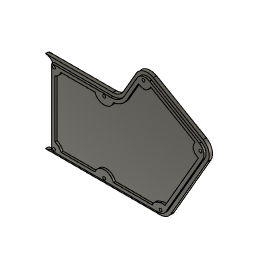
Barcode+scanner (Autodesk Fusion 360 design; units mm, degrees)
Autodesk Fusion 360 part; units mm, degrees
(part 1 of 5)
sketch "Sketch1" plane through (0, 0, 0) normal (0, 1, 0) x (1, 0, 0) in component "GM60 standalone"
  line L0 (0, 0) -> (165.7543, 0)
  line L1 (178.7446, -7.5) -> (207.1218, -56.6506)
  line L2 (201.6314, -77.141) -> (166.9904, -97.141)
  line L3 (146.5, -91.6506) -> (138.3301, -77.5)
  line L4 (125.3397, -70) -> (19, -70)
  line L5 (4, -85) -> (4, -112)
  line L6 (1, -115) -> (0, -115)
  line L7 (0, -115) -> (0, 0)
  arc A0 (178.7446, -7.5) -> (165.7543, 0) centre (165.7543, -15) ccw
  arc A1 (201.6314, -77.141) -> (207.1218, -56.6506) centre (194.1314, -64.1506) ccw
  arc A2 (146.5, -91.6506) -> (166.9904, -97.141) centre (159.4904, -84.1506) ccw
  arc A3 (138.3301, -77.5) -> (125.3397, -70) centre (125.3397, -85) ccw
  arc A4 (19, -70) -> (4, -85) centre (19, -85) ccw
  line L8 (4, -4) -> (165.7543, -4)
  arc A5 (175.2805, -9.5) -> (165.7543, -4) centre (165.7543, -15) ccw
  line L9 (175.2805, -9.5) -> (203.6577, -58.6506)
  arc A6 (199.6314, -73.6769) -> (203.6577, -58.6506) centre (194.1314, -64.1506) ccw
  line L10 (199.6314, -73.6769) -> (164.9904, -93.6769)
  arc A7 (149.9641, -89.6506) -> (164.9904, -93.6769) centre (159.4904, -84.1506) ccw
  line L11 (149.9641, -89.6506) -> (141.7942, -75.5)
  arc A8 (141.7942, -75.5) -> (125.3397, -66) centre (125.3397, -85) ccw
  line L12 (125.3397, -66) -> (19, -66)
  arc A9 (19, -66) -> (4, -73.3381) centre (19, -85) ccw
  line L13 (4, -73.3381) -> (4, -4)
  arc A10 (1, -115) -> (4, -112) centre (1, -112) ccw
  arc A11 (4, -14) -> (14, -4) centre (4, -4) ccw
  line L14 (4, -4) -> (11.0711, -11.0711) construction
  circle A12 centre (7.5355, -7.5355) radius 2
  line L15 (19, -85) -> (19, -51) construction
  arc A13 (4, -51) -> (19, -66) centre (19, -51) ccw
  line L16 (19, -66) -> (4, -66) construction
  circle A14 centre (7, -66) radius 2
  line L17 (159.4904, -84.1506) -> (154, -104.641) construction
  spline S0 degree 2 poles (149.9641, -89.6506) (159.4904, -84.1506) (164.9904, -93.6769) knots 0 0 0 1.944544 1.944544 1.944544 weights 1 3 1
  circle A15 centre (157.6786, -90.9121) radius 2
  line L18 (175.2805, -9.5) -> (172.1601, -11.3016)
  line L19 (162.6789, -4) -> (162.6789, -6.8969)
  line L20 (164.656, -9.7171) -> (169.6373, -11.5237)
  arc A16 (162.6789, -6.8969) -> (164.656, -9.7171) centre (165.6789, -6.8969) ccw
  arc A17 (169.6373, -11.5237) -> (172.1601, -11.3016) centre (170.6601, -8.7035) ccw
  spline S1 degree 2 poles (199.6314, -73.6769) (194.1314, -64.1506) (203.6577, -58.6506) knots 0 0 0 1.944543 1.944543 1.944543 weights 1 3 1
  line L21 (194.1314, -64.1506) -> (214.6218, -69.641) construction
  circle A18 centre (200.8929, -65.9624) radius 2
  line L22 (162.6789, -4) -> (175.2805, -9.5) construction
  arc A19 (125.3397, -66) -> (109.3397, -66) centre (117.3397, -66) ccw
  line L23 (117.3397, -66) -> (117.3397, -58) construction
  circle A20 centre (117.3397, -62) radius 2
  line L24 (4, -85) -> (0, -85)
  line L25 (168.9797, -6.75) -> (167.1467, -10.6204) construction
  circle A21 centre (168.5515, -7.6542) radius 2
  circle A22 centre (7.5355, -7.5355) radius 2.25
  circle A23 centre (168.5515, -7.6542) radius 2.25
  circle A24 centre (200.8929, -65.9624) radius 2.25
  circle A25 centre (117.3397, -62) radius 2.25
  circle A26 centre (7, -66) radius 2.25
  circle A27 centre (157.6786, -90.9121) radius 2.25
  line L26 (4, -38.669) -> (192.1213, -38.669) construction
  line L27 (157, -6.669) -> (87, -6.669)
  line L28 (87, -6.669) -> (87, -56.669)
  line L29 (87, -56.669) -> (157, -56.669)
  line L30 (157, -56.669) -> (157, -6.669)
  line L31 (157, -6.669) -> (87, -56.669) construction
  line L32 (87, -6.669) -> (157, -56.669) construction
  line L33 (155.04, -8.604) -> (88.96, -8.604)
  line L34 (88.96, -8.604) -> (88.96, -54.734) construction
  line L35 (88.96, -54.734) -> (155.04, -54.734) construction
  line L36 (155.04, -54.734) -> (155.04, -8.604) construction
  line L37 (155.04, -8.604) -> (88.96, -54.734) construction
  line L38 (88.96, -8.604) -> (155.04, -54.734) construction
  circle A28 centre (88.96, -54.734) radius 0.95
  circle A29 centre (88.96, -54.734) radius 3.45
  circle A30 centre (155.04, -54.734) radius 0.95
  circle A31 centre (155.04, -54.734) radius 3.45
  circle A32 centre (155.04, -8.604) radius 0.95
  circle A33 centre (155.04, -8.604) radius 3.45
  circle A34 centre (88.96, -8.604) radius 3.45
  circle A35 centre (88.96, -8.604) radius 0.95
  point P0 (214.6218, -69.641)
  point P1 (154, -104.641)
  point P2 (134, -70)
  point P3 (4, -70)
  point P4 (4, -115)
  point P5 (170.9504, -12)
  point P6 (162.6789, -9)
  point P7 (122, -31.669)
  point P8 (122, -31.669)
  point P9 (122, -31.669)
  dimension "d1" = 130
  dimension "d2" = 70
  dimension "d3" = 70
  dimension "d4" = 40
  dimension "d5" = 4
  dimension "d7" = 45
  dimension "d8" = 120
  dimension "d9" = 4
  dimension "d40" = 15
  dimension "d47" = 3
  dimension "d84" = 10
  dimension "d85" = 4
  dimension "d88" = 19
  dimension "d94" = 15
  dimension "d95" = 19
  dimension "d96" = 15
  dimension "d97" = 15
  dimension "d98" = 3
  dimension "d101" = 11
  dimension "d102" = 15
  dimension "d105" = 7
  dimension "d111" = 5
  dimension "d112" = 5
  dimension "d113" = 3
  dimension "d115" = 7
  dimension "d120" = 8
  dimension "d121" = 8
  dimension "d139" = 1
  dimension "d147" = 0.25
  dimension "d148" = 0.25
  dimension "d149" = 0.25
  dimension "d150" = 0.25
  dimension "d151" = 0.25
  dimension "d153" = 3.2821
  dimension "d157" = 0.25
  dimension "d234" = 70
  dimension "d235" = 50
  dimension "d236" = 66.08
  dimension "d237" = 46.13
  dimension "d238" = 1.9
  dimension "d239" = 2.5
  dimension "d240" = 7
  dimension "d241" = 118
  constraint coincident L0.start L7.end
  constraint horizontal L0
  constraint perpendicular L1 L2
  constraint parallel L0 L4
  constraint perpendicular L4 L5
  constraint parallel L1 L3
  constraint perpendicular L5 L6
  constraint perpendicular L0 L7
  constraint tangent L0 A0
  constraint tangent L1 A0
  constraint coincident P0 L1
  constraint coincident P0 L2
  constraint tangent L1 A1
  constraint tangent L2 A1
  constraint equal A0 A1
  constraint coincident P1 L2
  constraint coincident P1 L3
  constraint tangent L2 A2
  constraint tangent L3 A2
  constraint equal A0 A2
  constraint coincident P2 L3
  constraint coincident P2 L4
  constraint tangent L3 A3
  constraint tangent L4 A3
  constraint equal A0 A3
  constraint coincident P3 L4
  constraint coincident P3 L5
  constraint tangent L4 A4
  constraint tangent L5 A4
  constraint equal A0 A4
  constraint coincident P4 L5
  constraint coincident P4 L6
  constraint tangent L5 A10
  constraint tangent L6 A10
  constraint coincident L13 A11.start
  constraint coincident L8 A11.end
  constraint coincident L8.start L13.end
  constraint midpoint A11 L14.end
  constraint midpoint L14 A12.centre
  constraint coincident A4.centre A9.centre
  constraint perpendicular L12 L15
  constraint coincident L13 A13.start
  constraint coincident L15.end A13.centre
  constraint coincident L13 L16.end
  constraint tangent A9 L16
  constraint perpendicular L13 L16
  constraint coincident L16 A14.centre
  constraint equal A12 A14
  constraint coincident A2.centre A7.centre
  constraint coincident P1 L17.end
  constraint coincident L17 A15.centre
  constraint equal A12 A15
  constraint perpendicular L9 L18
  constraint coincident L8 L19.start
  constraint perpendicular L8 L19
  constraint coincident P6 L19
  constraint coincident P6 L20
  constraint tangent L19 A16
  constraint tangent L20 A16
  constraint coincident P5 L20
  constraint coincident P5 L18
  constraint tangent L20 A17
  constraint tangent L18 A17
  constraint equal A16 A17
  constraint coincident A1.centre A6.centre
  constraint coincident P0 L21.end
  constraint coincident L21 A18.centre
  constraint equal A12 A18
  constraint coincident L12 A8.end
  constraint coincident L12 A19.centre
  constraint coincident A19.centre L23.start
  constraint perpendicular L12 L23
  constraint midpoint L23 A20.centre
  constraint equal A12 A20
  constraint coincident L7 L24.end
  constraint perpendicular L7 L24
  constraint midpoint L22 L25.start
  constraint midpoint L20 L25.end
  constraint coincident L25 A21.centre
  constraint equal A12 A21
  constraint midpoint L13 L26.start
  constraint coincident L9 L26.end
  constraint perpendicular L13 L26
  constraint horizontal L27
  constraint perpendicular L27 L28
  constraint parallel L27 L29
  constraint parallel L28 L30
  constraint coincident L31 P9
  constraint coincident L32 P9
  constraint coincident P9 P8
  constraint horizontal L33
  constraint perpendicular L33 L34
  constraint parallel L33 L35
  constraint parallel L34 L36
  constraint coincident L37 P9
  constraint coincident L38 P9
  constraint coincident L34.end L35.start
  constraint coincident L35.end L36.start
  constraint coincident L33.start L36.end
  constraint concentric A32 A33
  constraint coincident L33.end L34.start
  constraint concentric A34 A35
  constraint equal A29 A31
  constraint equal A31 A33
  constraint equal A33 A34
  constraint equal A28 A32
  constraint equal A30 A32
  constraint equal A30 A35
  measures "d1" distance of P2 P3
  measures "d2" distance of L0 L4
  measures "d3" distance of P0 P1
  measures "d4" distance of P1 P2
  measures "d5" distance of P4 L6.end
  measures "d7" distance of P3 P4
  measures "d8" angle of L3 L4
  measures "d40" radius of A0
  measures "d47" radius of A10
  measures "d84" radius of A11
  measures "d85" diameter of A12
  measures "d88" radius of A9
  measures "d94" distance of L4.end A4.centre
  measures "d95" distance of A4.centre L12
  measures "d96" distance of L5.start A4.centre
  measures "d97" distance of L12.end L15.end
  measures "d98" distance of L13 A14.centre
  measures "d101" radius of A7
  measures "d102" radius of A2
  measures "d105" distance of A2.centre A15.centre
  measures "d111" distance of L19.start P6
  measures "d112" distance of A5.start P5
  measures "d113" radius of A16
  measures "d115" distance of A1.centre A18.centre
  measures "d120" radius of A19
  measures "d121" distance of A8.end A19.centre
  measures "d139" distance of L22 A21.centre
  measures "d153" distance of L25.end A21.centre
  measures "d234" distance of L28.end L29.end
  measures "d235" distance of L27.end L28.end
  measures "d236" distance of L34.end L35.end
  measures "d237" distance of L33.end L34.end
  measures "d238" diameter of A28
  measures "d240" distance of L26 P9
  measures "d241" distance of L13 P9
extrude "Extrude1" add sketch "Sketch1" along normal blind 60 contours L0 L1 L2 L3 L4 L7 A0 A1 A2 A3 A4 L24 | L5 L6 L7 A10 L24 picked at (59.9181, -1.3333) picked at (1.3333, -104) makes body 1 in component "GM60 standalone"
sketch "Display cutout" plane through (81.8109, 0, 141.7006) normal (-0.5, 0, -0.866025) x (0, -1, 0) in component "GM60 standalone"
  line L0 (0, -136.0474) -> (0, -96.0474)
  line L1 (-60, -96.0474) -> (-60, -136.0474)
  line L2 (0, -116.0474) -> (-60, -116.0474) construction
  line L3 (0, -96.0474) -> (-60, -96.0474)
  line L4 (-60, -136.0474) -> (0, -136.0474)
  line L5 (-38.325, -103.0474) -> (-38.325, -108.5474)
  line L6 (-43.825, -123.5474) -> (-43.825, -132.5474)
  line L7 (-43.825, -103.0474) -> (-16.175, -103.0474)
  line L8 (-43.825, -132.5474) -> (-43.825, -127.8474)
  line L9 (-43.825, -132.5474) -> (-16.175, -132.5474)
  line L10 (-38.325, -132.5474) -> (-43.825, -132.5474)
  line L11 (-43.825, -127.8474) -> (-38.325, -127.8474)
  line L12 (-38.325, -127.8474) -> (-38.325, -132.5474)
  line L13 (-43.825, -108.5474) -> (-43.825, -103.0474)
  line L14 (-43.825, -108.5474) -> (-43.825, -123.5474)
  line L15 (-16.175, -123.5474) -> (-16.175, -108.5474)
  line L16 (-21.675, -132.5474) -> (-21.675, -127.8474)
  line L17 (-43.825, -123.5474) -> (-16.175, -108.5474) construction
  line L18 (-16.175, -103.0474) -> (-16.175, -108.5474)
  line L19 (-16.175, -132.5474) -> (-16.175, -123.5474)
  line L20 (-21.675, -127.8474) -> (-16.175, -127.8474)
  line L21 (-16.175, -127.8474) -> (-16.175, -132.5474)
  line L22 (-16.175, -108.5474) -> (-43.825, -108.5474)
  line L23 (-16.175, -123.5474) -> (-43.825, -123.5474)
  line L24 (-43.825, -123.5474) -> (-16.175, -123.5474)
  line L25 (-16.175, -108.5474) -> (-43.825, -108.5474)
  line L26 (-21.675, -103.0474) -> (-21.675, -108.5474)
  line L27 (-16.175, -123.5474) -> (-43.825, -108.5474) construction
  line L28 (-16.175, -132.5474) -> (-21.675, -132.5474)
  point P0 (-30, -116.0474)
  point P1 (-30, -116.0474)
  point P2 (-30, -116.0474)
  dimension "d64" = 27.65
  dimension "d65" = 15
  dimension "d66" = 5.5
  dimension "d67" = 9
  dimension "d68" = 5.5
  dimension "d69" = 5.5
  dimension "d70" = 4.7
  dimension "d225" = 29.5
  dimension "d226" = 24.8
  constraint midpoint L0 L2.start
  constraint midpoint L1 L2.end
  constraint horizontal L24
  constraint perpendicular L15 L24
  constraint parallel L24 L25
  constraint parallel L14 L15
  constraint coincident P2 L17
  constraint coincident P2 L27
  constraint perpendicular L13 L22
  constraint parallel L7 L22
  constraint parallel L13 L18
  constraint perpendicular L6 L23
  constraint parallel L9 L23
  constraint parallel L6 L19
  constraint coincident L26.start L7
  constraint coincident L26.end L25
  constraint perpendicular L25 L26
  constraint coincident L5.start L7
  constraint coincident L5.end L22
  constraint perpendicular L5 L22
  constraint horizontal L28
  constraint vertical L16
  constraint horizontal L20
  constraint vertical L21
  constraint collinear L16 L26
  constraint horizontal L10
  constraint vertical L8
  constraint horizontal L11
  constraint vertical L12
  constraint coincident L8.end L6
  constraint coincident L10.start L9
  constraint collinear L5 L12
  constraint collinear L11 L20
  constraint coincident P2 P1
  constraint midpoint L2 P2
  measures "d64" distance of L15.end L13.start
  measures "d65" distance of L15.end L15.start
  measures "d66" distance of L15.end L7.end
  measures "d67" distance of L15.start L9.end
  measures "d68" distance of L18 L26
  measures "d69" distance of L5 L13
  measures "d70" distance of L20 L28
  measures "d225" distance of L7 L9
  measures "d226" distance of L7 L20
sketch "Sketch1 (2)" plane through (0, 0, 0) normal (0, 0, 1) x (1, 0, 0) in component "Sample display"
  line L0 (9.6502, -9.1979) -> (15.1502, -9.1979)
  line L1 (-12.4998, -13.8979) -> (-12.4998, -9.1979)
  line L2 (-12.4998, 10.1021) -> (-12.4998, 15.6021)
  line L3 (-6.9998, -9.1979) -> (-6.9998, -13.8979)
  line L4 (15.1502, -4.8979) -> (-12.4998, -4.8979)
  line L5 (-12.4998, -4.8979) -> (15.1502, 10.1021) construction
  line L6 (9.6502, -13.8979) -> (9.6502, -9.1979)
  line L7 (-6.9998, 15.6021) -> (-6.9998, 10.1021)
  line L8 (-6.9998, -13.8979) -> (-12.4998, -13.8979)
  line L9 (-12.4998, -4.8979) -> (-12.4998, -13.8979)
  line L10 (9.6502, 15.6021) -> (9.6502, 10.1021)
  line L11 (15.1502, -4.8979) -> (15.1502, 10.1021)
  line L12 (15.1502, 10.1021) -> (-12.4998, 10.1021)
  line L13 (15.1502, -13.8979) -> (15.1502, -4.8979)
  line L14 (-12.4998, -9.1979) -> (-6.9998, -9.1979)
  line L15 (15.1502, -13.8979) -> (9.6502, -13.8979)
  line L16 (15.1502, 10.1021) -> (-12.4998, 10.1021)
  line L17 (-12.4998, -13.8979) -> (15.1502, -13.8979)
  line L18 (-12.4998, -4.8979) -> (15.1502, -4.8979)
  line L19 (15.1502, -9.1979) -> (15.1502, -13.8979)
  line L20 (15.1502, 15.6021) -> (15.1502, 10.1021)
  line L21 (15.1502, -4.8979) -> (-12.4998, 10.1021) construction
  line L22 (-12.4998, 10.1021) -> (-12.4998, -4.8979)
  line L23 (30, 0.866) -> (-30, 0.866) construction
  line L24 (-12.4998, 15.6021) -> (15.1502, 15.6021)
  line L25 (21.1502, -19.8979) -> (-18.4998, -19.8979)
  line L26 (-18.4998, -19.8979) -> (-18.4998, 21.6021)
  line L27 (-18.4998, 21.6021) -> (21.1502, 21.6021)
  line L28 (21.1502, 21.6021) -> (21.1502, -19.8979)
  line L29 (21.1502, -19.8979) -> (-18.4998, 21.6021) construction
  line L30 (-18.4998, -19.8979) -> (21.1502, 21.6021) construction
  point P0 (1.3252, 2.6021)
  point P1 (1.3252, 0.8521)
  point P2 (1.3252, 2.6021)
  point P3 (0, 0.866)
  point P4 (1.3252, 0.8521)
  dimension "d202" = 27.65
  dimension "d203" = 15
  dimension "d204" = 5.5
  dimension "d205" = 9
  dimension "d206" = 5.5
  dimension "d207" = 5.5
  dimension "d208" = 4.7
  dimension "d211" = 6
  dimension "d212" = 6
  dimension "d213" = 6
  dimension "d214" = 6
  dimension "d221" = 29.5
  dimension "d224" = 24.8
  constraint coincident P3 L23
  constraint midpoint P3 L23
  constraint horizontal L18
  constraint perpendicular L11 L18
  constraint parallel L12 L18
  constraint parallel L11 L22
  constraint coincident P2 L5
  constraint coincident P2 L21
  constraint perpendicular L2 L16
  constraint parallel L16 L24
  constraint parallel L2 L20
  constraint perpendicular L4 L9
  constraint parallel L4 L17
  constraint parallel L9 L13
  constraint coincident L10.start L24
  constraint coincident L10.end L12
  constraint perpendicular L10 L12
  constraint coincident L7.start L24
  constraint coincident L7.end L16
  constraint perpendicular L7 L16
  constraint horizontal L15
  constraint vertical L6
  constraint horizontal L0
  constraint vertical L19
  constraint collinear L6 L10
  constraint horizontal L8
  constraint vertical L1
  constraint horizontal L14
  constraint vertical L3
  constraint coincident L1.end L9
  constraint coincident L3.end L17
  constraint collinear L3 L7
  constraint collinear L0 L14
  constraint coincident P2 P0
  constraint horizontal L25
  constraint perpendicular L25 L26
  constraint parallel L25 L27
  constraint parallel L26 L28
  constraint coincident L29 P4
  constraint coincident L30 P4
  constraint coincident P4 P1
  measures "d202" distance of L5.end L2.start
  measures "d203" distance of L5.end L4.start
  measures "d204" distance of L5.end L20.start
  measures "d205" distance of L13.start L4.start
  measures "d206" distance of L10 L20
  measures "d207" distance of L2 L7
  measures "d208" distance of L0 L15
  measures "d211" distance of L24 L27
  measures "d212" distance of L22 L26
  measures "d213" distance of L11 L28
  measures "d214" distance of L17 L25
  measures "d221" distance of L17 L24
  measures "d224" distance of L14 L24
extrude "Extrude1'" add sketch "Sketch1 (2)" along normal blind 4 separate body contours L25 L26 L27 L28 picked at (19.1502, -1.0645) makes body 2 in component "Sample display"
extrude "Extrude2" add sketch "Sketch1 (2)" along normal blind 0.6 contours L0 L3 L4 L6 L9 L13 L14 L17 L18 | L7 L10 L12 L16 L24 picked at (-1.4498, -6.3312) picked at (-1.4498, 13.7688) bodies 2 in component "Sample display"
extrude "Extrude3" add sketch "Sketch1 (2)" along normal blind 2 contours L0 L6 L13 L15 L17 L19 | L1 L3 L8 L9 L14 L17 | L10 L12 L16 L20 L24 | L2 L7 L12 L16 L24 picked at (13.3168, -10.7645) picked at (-8.8332, -10.7645) picked at (13.3168, 11.9355) picked at (-10.6665, 13.7688) bodies 2 in component "Sample display"
fillet "Fillet1" radius 15 4 edges at (-18.4998, 21.6021, 2) (21.1502, 21.6021, 2) (-18.4998, -19.8979, 2) (21.1502, -19.8979, 2) on bodies 2 in component "Sample display"
extrude "Extrude8" add sketch "Sketch1" against normal blind 4 contours L0 L1 L2 L3 L4 L7 A0 A1 A2 A3 A4 L24 | L5 L6 L7 A10 L24 | L8 L13 A11 | L8 L9 L10 L11 A8 L12 L13 A11 A13 S0 L18 L19 L20 A16 A17 S1 A19 | L8 A5 L18 L19 L20 A16 A17 | A9 L13 A13 | L12 A19 | A6 S1 | A7 S0 | A12 | A14 | A15 | A18 | A20 | A21 | A22 | A23 | A24 | A25 | A26 | A27 | L27 L30 A33 | L27 L30 A33 | L27 L33 A33 A34 | L28 L29 L30 L33 A29 A31 A33 A34 | L27 L28 A34 | L27 L28 A34 | L29 L30 A31 | L29 L30 A31 | L28 L29 A29 | L28 L29 A29 | A28 | A30 | A32 | A35 picked at (59.9181, -1.3333) picked at (1.3333, -104) picked at (4.4369, -8.6236) picked at (39.1305, -42.8013) picked at (172.3644, -9.3579) picked at (11.2568, -65.9119) picked at (117.2837, -65.4146) picked at (198.6139, -69.7182) picked at (153.9527, -88.5857) picked at (6.8451, -7.203) picked at (6.363, -67.1034) picked at (158.3157, -92.0155) picked at (201.5299, -67.0658) picked at (116.4591, -62.4828) picked at (168.3942, -8.8468) picked at (9.6938, -7.6473) picked at (170.7098, -7.766) picked at (198.7346, -66.0742) picked at (118.0242, -64.0499) picked at (7.0498, -68.1606) picked at (155.7826, -89.875) picked at (156.6598, -8.9526) picked at (153.8961, -6.5342) picked at (131.8633, -8.2629) picked at (132.0458, -38.7358) picked at (87.3402, -8.9526) picked at (90.1066, -6.5371) picked at (153.8961, -56.8039) picked at (156.6598, -54.3855) picked at (87.3402, -54.3855) picked at (90.1066, -56.801) picked at (89.1921, -54.9494) picked at (155.3016, -54.8305) picked at (155.3253, -8.7414) picked at (88.7279, -8.9138) bodies 1 in component "GM60 standalone"
sketch "Sensor cutout" plane through (0, 0, 66) normal (0, 0, -1) x (1, 0, 0) in component "GM60 standalone"
  line L0 (125.3397, 0) -> (19, 0)
  line L1 (19, 0) -> (19, -60)
  line L2 (19, -60) -> (125.3397, -60)
  line L3 (125.3397, -60) -> (125.3397, 0)
  line L4 (19, -30) -> (125.3397, -30) construction
  circle A0 centre (69, -30) radius 13
  dimension "d48" = 26
  dimension "d49" = 50
  constraint midpoint L1 L4.start
  constraint coincident L4 A0.centre
  measures "d48" diameter of A0
  measures "d49" distance of L4.start A0.centre
extrude "Extrude1''" cut sketch "Sensor cutout" against normal up to surface (4 mm away) contours A0 picked at (73.0967, -26.8426) bodies 1 in component "GM60 standalone"
sketch "Power cutout" plane through (0, 0, 4) normal (0, 0, 1) x (-1, 0, 0) in component "GM60 standalone"
  line L0 (-4, 0) -> (-165.7543, 0)
  line L1 (-165.7543, 0) -> (-165.7543, -60)
  line L2 (-165.7543, -60) -> (-4, -60)
  line L3 (-4, -60) -> (-4, 0)
  line L4 (-4, -30) -> (-165.7543, -30) construction
  circle A0 centre (-34, -30) radius 4
  line L5 (-38.95, -32.8579) -> (-34, -35.7158)
  line L6 (-34, -35.7158) -> (-29.05, -32.8579)
  line L7 (-29.05, -32.8579) -> (-29.05, -27.1421)
  line L8 (-29.05, -27.1421) -> (-34, -24.2842)
  line L9 (-34, -24.2842) -> (-38.95, -27.1421)
  line L10 (-38.95, -27.1421) -> (-38.95, -32.8579)
  line L11 (-102.7993, -29.1827) -> (-102.7993, -29)
  circle A1 centre (-79, -30) radius 4.625
  circle A2 centre (-79, -30) radius 2.25
  circle A3 centre (-79, -30) radius 7.625
  point P0 (-34, -30)
  dimension "d52" = 8
  dimension "d53" = 30
  dimension "d133" = 9.9
  dimension "d191" = 3
  dimension "d193" = 9.25
  dimension "d194" = 4.5
  dimension "d195" = 75
  constraint midpoint L3 L4.start
  constraint midpoint L1 L4.end
  constraint coincident L4 P0
  constraint coincident P0 A0.centre
  constraint concentric A1 A2
  constraint coincident L4 A1.centre
  measures "d52" diameter of A0
  measures "d53" distance of L3 P0
  measures "d133" distance of L7 L10
  measures "d193" diameter of A1
  measures "d194" diameter of A2
  measures "d195" distance of L3 A1.centre
extrude "Extrude2'" cut sketch "Power cutout" against normal up to surface (4 mm away) contours A0 picked at (-34.787, -30.4507) bodies 1 in component "GM60 standalone"
sketch "Sketch1 (3)" plane through (0, 60, 0) normal (0, 1, 0) x (-1, 0, 0) in component "LID"
  arc A0 (-149.9641, 89.6506) -> (-164.9904, 93.6769) centre (-159.4904, 84.1506) ccw
  line L0 (-149.9641, 89.6506) -> (-141.7942, 75.5)
  arc A1 (-141.7942, 75.5) -> (-125.3397, 66) centre (-125.3397, 85) ccw
  line L1 (-125.3397, 66) -> (-19, 66)
  arc A2 (-19, 66) -> (-4, 73.3381) centre (-19, 85) ccw
  line L2 (-4, 73.3381) -> (-4, 4)
  line L3 (-4, 4) -> (-165.7543, 4)
  line L4 (-175.2805, 9.5) -> (-203.6577, 58.6506)
  arc A3 (-199.6314, 73.6769) -> (-203.6577, 58.6506) centre (-194.1314, 64.1506) ccw
  line L5 (-199.6314, 73.6769) -> (-164.9904, 93.6769)
  line L6 (0, 115) -> (-1, 115)
  arc A4 (-1, 115) -> (-4, 112) centre (-1, 112) ccw
  line L7 (-4, 112) -> (-4, 85)
  arc A5 (-19, 70) -> (-4, 85) centre (-19, 85) ccw
  line L8 (-19, 70) -> (-125.3397, 70)
  arc A6 (-138.3301, 77.5) -> (-125.3397, 70) centre (-125.3397, 85) ccw
  line L9 (-138.3301, 77.5) -> (-146.5, 91.6506)
  arc A7 (-146.5, 91.6506) -> (-166.9904, 97.141) centre (-159.4904, 84.1506) ccw
  line L10 (-166.9904, 97.141) -> (-201.6314, 77.141)
  arc A8 (-201.6314, 77.141) -> (-207.1218, 56.6506) centre (-194.1314, 64.1506) ccw
  line L11 (-207.1218, 56.6506) -> (-178.7446, 7.5)
  arc A9 (-178.7446, 7.5) -> (-165.7543, 0) centre (-165.7543, 15) ccw
  line L12 (-165.7543, 0) -> (0, 0)
  line L13 (0, 0) -> (0, 115)
  circle A10 centre (-7, 66) radius 1.75
  circle A11 centre (-7.5355, 7.5355) radius 1.75
  circle A12 centre (-200.8929, 65.9624) radius 1.75
  circle A13 centre (-157.6786, 90.9121) radius 1.75
  circle A14 centre (-117.3397, 62) radius 1.75
  line L14 (-4, 85) -> (0, 85)
  arc A15 (-175.2805, 9.5) -> (-165.7543, 4) centre (-165.7543, 15) ccw
  circle A16 centre (-168.5515, 7.6542) radius 1.75
  circle A17 centre (-200.8929, 65.9624) radius 2.75
  circle A18 centre (-157.6786, 90.9121) radius 2.75
  circle A19 centre (-117.3397, 62) radius 2.75
  circle A20 centre (-7, 66) radius 2.75
  circle A21 centre (-168.5515, 7.6542) radius 2.75
  circle A22 centre (-7.5355, 7.5355) radius 2.75
  point P0 (-7.5355, 7.5355)
  point P1 (-7, 66)
  point P2 (-200.8929, 65.9624)
  point P3 (-157.6786, 90.9121)
  point P4 (-117.3397, 62)
  point P5 (-168.5515, 7.6542)
  dimension "d116" = 3.5
  dimension "d140" = 5.5
  constraint coincident P1 A10.centre
  constraint coincident P0 A11.centre
  constraint coincident P2 A12.centre
  constraint coincident P3 A13.centre
  constraint equal A10 A11
  constraint equal A12 A13
  constraint coincident P4 A14.centre
  constraint equal A11 A14
  constraint coincident P5 A16.centre
  constraint equal A11 A16
  constraint concentric A13 A18
  constraint concentric A14 A19
  constraint concentric A10 A20
  constraint concentric A16 A21
  constraint concentric A11 A22
  constraint equal A21 A22
  constraint equal A17 A21
  constraint equal A17 A18
  constraint equal A18 A19
  constraint equal A19 A20
  measures "d116" diameter of A11
  measures "d140" diameter of A22
extrude "Extrude1'''" add sketch "Sketch1 (3)" along normal blind 4 separate body contours A0 L0 A1 L1 A2 L2 L3 L4 A3 L5 A15 | A5 L8 A6 L9 A7 L10 A8 L11 A9 L12 L13 L14 | A10 | A11 | A12 | A13 | A14 | A16 | A17 | A18 | A19 | A20 | A21 | A22 picked at (-97.465, 23.3568) picked at (-1.3333, 52.7794) picked at (-7.482, 65.4975) picked at (-7.1398, 7.5073) picked at (-200.9394, 66.5054) picked at (-157.7251, 91.4551) picked at (-116.976, 62.63) picked at (-169.3367, 8.1738) picked at (-201.2952, 63.5859) picked at (-158.0809, 88.5356) picked at (-114.9333, 61.8634) picked at (-9.2592, 65.1601) picked at (-168.9538, 5.2777) picked at (-5.1356, 7.312) makes body 3 in component "LID"
extrude "Extrude2''" add sketch "Sketch1 (3)" against normal blind 2.5 contours A0 L0 A1 L1 A2 L2 L3 L4 A3 L5 A15 | A17 | A18 | A19 | A20 | A21 | A22 picked at (-97.465, 23.3568) picked at (-201.2952, 63.5859) picked at (-158.0809, 88.5356) picked at (-114.9333, 61.8634) picked at (-9.2592, 65.1601) picked at (-168.9538, 5.2777) picked at (-5.1356, 7.312) bodies 3 in component "LID"
extrude "Extrude3'" cut sketch "Display cutout" against normal up to surface (4 mm away) contours L14 L15 L22 L23 L24 L25 picked at (-27.225, -118.5474) bodies 1 in component "GM60 standalone"
extrude "Extrude4" cut sketch "Display cutout" against normal blind 2 contours L5 L7 L13 L22 L25 | L7 L18 L22 L25 L26 | L6 L8 L9 L10 L11 L12 | L9 L16 L19 L20 L21 L28 picked at (-41.9917, -106.7141) picked at (-19.8417, -104.8807) picked at (-40.1583, -129.4141) picked at (-18.0083, -129.4141) bodies 1 in component "GM60 standalone"
extrude "Extrude5" cut sketch "Display cutout" against normal blind 3.4 contours L5 L7 L22 L25 L26 | L6 L9 L11 L12 L16 L19 L20 L23 L24 picked at (-27.225, -106.7141) picked at (-32.775, -124.9807) bodies 1 in component "GM60 standalone"
extrude "Extrude7" add sketch "Sketch1" along normal up to surface (57.25 mm away) contours L8 L13 A11 | L8 A5 L18 L19 L20 A16 A17 | A9 L13 A13 | L12 A19 | A6 S1 | A7 S0 | A22 | A23 | A24 | A25 | A26 | A27 picked at (4.4369, -8.6236) picked at (172.3644, -9.3579) picked at (11.2568, -65.9119) picked at (117.2837, -65.4146) picked at (198.6139, -69.7182) picked at (153.9527, -88.5857) picked at (9.6938, -7.6473) picked at (170.7098, -7.766) picked at (198.7346, -66.0742) picked at (118.0242, -64.0499) picked at (7.0498, -68.1606) picked at (155.7826, -89.875) bodies 1 in component "GM60 standalone"
extrude "Extrude3''" cut sketch "Sketch1 (3)" against normal up to surface (6.5 mm away) from surface at 4 contours A10 | A11 | A12 | A13 | A14 | A16 picked at (-7.482, 65.4975) picked at (-7.1398, 7.5073) picked at (-200.9394, 66.5054) picked at (-157.7251, 91.4551) picked at (-116.976, 62.63) picked at (-169.3367, 8.1738) bodies 3 in component "LID"
extrude "Extrude8'" add sketch "Sketch1" along normal blind 4 from surface at 60 contours L5 L6 L7 A10 L24 picked at (1.3333, -104) bodies 1 in component "GM60 standalone"
sketch "Sketch2" plane through (0, 0, 85) normal (0, 0, 1) x (-1, 0, 0) in component "LID"
  line L0 (0, -60) -> (-4, -60)
  line L1 (-4, -60) -> (-4, -64)
  line L2 (-4, -64) -> (0, -64)
  line L3 (0, -64) -> (0, -60)
  line L4 (0, -62) -> (-4, -62)
  constraint midpoint L3 L4.start
  constraint midpoint L1 L4.end
extrude "Extrude11" cut sketch "Power cutout" along normal blind 1.5 from surface at -4 contours L5 L6 L7 L8 L9 L10 picked at (-31.6833, -25.9874) bodies 1 in component "GM60 standalone"
extrude "Extrude12" [suppressed] in component "GM60 standalone"
extrude "Extrude6" cut sketch "Sketch1 (3)" against normal blind 3 from surface at 4 contours A17 | A18 | A19 | A20 | A21 | A22 picked at (-201.2952, 63.5859) picked at (-158.0809, 88.5356) picked at (-114.9333, 61.8634) picked at (-9.2592, 65.1601) picked at (-168.9538, 5.2777) picked at (-5.1356, 7.312) bodies 3 in component "LID"
extrude "Extrude13" cut sketch "Sketch1" against normal blind 1.5 from surface at 57.25 contours A22 | A23 | A24 | A25 | A26 | A27 picked at (9.6938, -7.6473) picked at (170.7098, -7.766) picked at (198.7346, -66.0742) picked at (118.0242, -64.0499) picked at (7.0498, -68.1606) picked at (155.7826, -89.875) bodies 1 in component "GM60 standalone"
extrude "Extrude18" cut sketch "Power cutout" against normal up to surface (4 mm away) contours A2 picked at (-79.6446, -29.2447) bodies 1 in component "GM60 standalone"
extrude "Extrude19" cut sketch "Power cutout" against normal blind 2 contours A1 picked at (-75.1923, -30.3416) bodies 1 in component "GM60 standalone"
sketch "Button cutout" plane through (127.3468, 0, -73.5237) normal (-0.866025, 0, 0.5) x (0, -1, 0) in component "GM60 standalone"
  line L0 (0, 95.8675) -> (0, 152.6218)
  line L1 (0, 152.6218) -> (-57.25, 152.6218)
  line L2 (-57.25, 152.6218) -> (-60, 152.6218)
  line L3 (-60, 152.6218) -> (-60, 95.8675)
  line L4 (-60, 95.8675) -> (-57.25, 95.8675)
  line L5 (-57.25, 95.8675) -> (0, 95.8675)
  line L6 (-64, 123.2917) -> (-64, 136.282)
  line L7 (-64, 136.282) -> (-64, 152.6218)
  line L8 (-64, 167.6218) -> (-64, 152.6218)
  line L9 (-64, 70.1218) -> (-64, 123.2917)
  line L10 (0, 124.2446) -> (-64, 124.2446) construction
  line L11 (-32, 124.2446) -> (-32, 152.6218) construction
  circle A0 centre (-48, 124.2446) radius 6
  circle A1 centre (-16, 124.2446) radius 6
  circle A2 centre (-48, 124.2446) radius 8 construction
  circle A3 centre (-16, 124.2446) radius 8 construction
  dimension "d228" = 12
  dimension "d229" = 16
  dimension "d230" = 32
  dimension "d233" = 16
  constraint midpoint L0 L10.start
  constraint coincident L6 L10.end
  constraint perpendicular L6 L10
  constraint midpoint L10 L11.start
  constraint coincident L1 L11.end
  constraint perpendicular L1 L11
  constraint coincident L10 A0.centre
  constraint symmetric L11 A0 A1
  constraint concentric A0 A2
  constraint symmetric L11 A2 A3
  measures "d228" diameter of A0
  measures "d229" distance of L9 A0.centre
  measures "d230" distance of A0.centre A1.centre
  measures "d233" diameter of A2
extrude "Extrude21" cut sketch "Button cutout" against normal up to surface (4 mm away) contours A0 | A1 picked at (-47.0665, 126.8643) picked at (-16.8801, 128.1008) bodies 1 in component "GM60 standalone"
extrude "Extrude22" add sketch "Sketch1" along normal blind 3 contours L27 L30 A33 | L27 L30 A33 | L27 L28 A34 | L27 L28 A34 | L29 L30 A31 | L29 L30 A31 | L28 L29 A29 | L28 L29 A29 picked at (156.6598, -8.9526) picked at (153.8961, -6.5342) picked at (87.3402, -8.9526) picked at (90.1066, -6.5371) picked at (153.8961, -56.8039) picked at (156.6598, -54.3855) picked at (87.3402, -54.3855) picked at (90.1066, -56.801) bodies 1 in component "GM60 standalone"
fillet "Fillet6" radius 1.5 4 edges at (151.8235, 0, 53.4865) (85.7435, 0, 53.4865) (151.8235, 0, 7.3565) (85.7435, 0, 7.3565) on bodies 1 in component "GM60 standalone"
extrude "Extrude23" cut 4 faces at (155.3016, 0, 54.8305) (89.1921, 0, 54.9494) (155.2374, 0, 8.8516) (88.7279, 0, 8.9138) along direction (0, -1, 0) blind 2 on bodies 1 bodies 1 in component "GM60 standalone"
extrude "Extrude20" add sketch "Power cutout" along normal blind 2 contours A3 picked at (-72.4206, -30.6086) bodies 1 in component "GM60 standalone"
sketch "Sketch1 (4)" plane through (0, 0, 0) normal (1, 0, 0) x (0, 1, 0) in component "GM67"
  line L0 (13.75, -23.25) -> (-13.75, -23.25)
  line L1 (-13.75, -23.25) -> (-13.75, 23.25)
  line L2 (-13.75, 23.25) -> (13.75, 23.25)
  line L3 (13.75, 23.25) -> (13.75, -23.25)
  line L4 (13.75, -23.25) -> (-13.75, 23.25) construction
  line L5 (-13.75, -23.25) -> (13.75, 23.25) construction
  line L6 (0, 0) -> (0, 66.3796) construction
  line L7 (12.35, -9.25) -> (-12.35, -9.25) construction
  line L8 (-12.35, -9.25) -> (-12.35, 17.15) construction
  line L9 (-12.35, 17.15) -> (12.35, 17.15) construction
  line L10 (12.35, 17.15) -> (12.35, -9.25) construction
  line L11 (12.35, -9.25) -> (-12.35, 17.15) construction
  line L12 (-12.35, -9.25) -> (12.35, 17.15) construction
  circle A0 centre (-12.35, 17.15) radius 1.25
  circle A1 centre (12.35, 17.15) radius 1.25
  circle A2 centre (12.35, -9.25) radius 1.25
  circle A3 centre (-12.35, -9.25) radius 1.25
  line L13 (0, 0) -> (0, -40) construction
  line L14 (14, -15.75) -> (-14, -15.75)
  line L15 (-14, -15.75) -> (-14, -25.75)
  line L16 (-14, -25.75) -> (14, -25.75)
  line L17 (14, -25.75) -> (14, -15.75)
  line L18 (14, -15.75) -> (-14, -25.75) construction
  line L19 (-14, -15.75) -> (14, -25.75) construction
  line L20 (0, 0) -> (-67.8363, 0) construction
  line L21 (13.75, -23.25) -> (13.75, 23.25)
  line L22 (0, 0) -> (0, 40) construction
  line L23 (-14, 25.75) -> (14, 25.75)
  circle A4 centre (12.35, -17.15) radius 1.25
  line L24 (14, 15.75) -> (-14, 25.75) construction
  line L25 (13.75, 23.25) -> (-13.75, 23.25)
  line L26 (12.35, 9.25) -> (-12.35, 9.25) construction
  line L27 (12.35, 9.25) -> (-12.35, -17.15) construction
  line L28 (-12.35, -17.15) -> (12.35, -17.15) construction
  line L29 (-13.75, -23.25) -> (13.75, -23.25)
  line L30 (14, 15.75) -> (-14, 15.75)
  line L31 (-13.75, 23.25) -> (-13.75, -23.25)
  circle A5 centre (12.35, 9.25) radius 1.25
  line L32 (-14, 15.75) -> (-14, 25.75)
  line L33 (13.75, 23.25) -> (-13.75, -23.25) construction
  circle A6 centre (-12.35, -17.15) radius 1.25
  line L34 (-14, 15.75) -> (14, 25.75) construction
  line L35 (14, 25.75) -> (14, 15.75)
  line L36 (0, 0) -> (0, -66.3796) construction
  line L37 (-12.35, 9.25) -> (12.35, -17.15) construction
  line L38 (-13.75, 23.25) -> (13.75, -23.25) construction
  circle A7 centre (-12.35, 9.25) radius 1.25
  line L39 (12.35, -17.15) -> (12.35, 9.25) construction
  line L40 (-12.35, 9.25) -> (-12.35, -17.15) construction
  point P0 (0, 3.95)
  point P1 (0, -20.75)
  point P2 (0, -3.95)
  point P3 (0, 20.75)
  dimension "d280" = 27.5
  dimension "d281" = 46.5
  dimension "d282" = 24.7
  dimension "d283" = 26.4
  dimension "d284" = 6.1
  dimension "d285" = 2.5
  dimension "d288" = 28
  dimension "d289" = 10
  dimension "d290" = 2.5
  constraint horizontal L0
  constraint perpendicular L0 L1
  constraint parallel L0 L2
  constraint parallel L1 L3
  constraint coincident L4 L6.start
  constraint coincident L5 L6.start
  constraint coincident L6.start L13.start
  constraint parallel L3 L6
  constraint horizontal L7
  constraint perpendicular L7 L8
  constraint parallel L7 L9
  constraint parallel L8 L10
  constraint coincident L11 P0
  constraint coincident L12 P0
  constraint coincident L6 P0
  constraint coincident L8.end L9.start
  constraint coincident L9.end L10.start
  constraint coincident L7.start L10.end
  constraint coincident L7.end L8.start
  constraint equal A0 A1
  constraint equal A1 A2
  constraint equal A2 A3
  constraint parallel L6 L13
  constraint horizontal L14
  constraint perpendicular L14 L15
  constraint parallel L14 L16
  constraint parallel L15 L17
  constraint coincident L18 P1
  constraint coincident L19 P1
  constraint coincident L13 P1
  constraint horizontal L20
  constraint symmetric L6.start L20 L13.start
  constraint symmetric L0.start L20 L2.end
  constraint symmetric L0.end L20 L1.end
  constraint symmetric L1.end L20 L0.end
  constraint symmetric L2.end L20 L0.start
  constraint symmetric L6.end L20 L36.end
  constraint symmetric L7.start L20 L26.start
  constraint symmetric L7.end L20 L26.end
  constraint symmetric L8.end L20 L27.end
  constraint symmetric L9.end L20 A4.centre
  constraint symmetric P0 L20 P2
  constraint symmetric A0 L20 A6
  constraint symmetric A1 L20 A4
  constraint symmetric A2 L20 A5
  constraint symmetric A3 L20 A7
  constraint symmetric L13.end L20 L22.end
  constraint symmetric L14.start L20 L24.start
  constraint symmetric L14.end L20 L30.end
  constraint symmetric L15.end L20 L23.start
  constraint symmetric L16.end L20 L23.end
  constraint symmetric P1 L20 P3
  measures "d280" distance of L1.end L2.end
  measures "d281" distance of L0.end L1.end
  measures "d282" distance of L8.end L9.end
  measures "d283" distance of L7.end L8.end
  measures "d284" distance of L2 L9
  measures "d285" diameter of A0
  measures "d288" distance of L15.end L16.end
  measures "d289" distance of L14.end L15.end
  measures "d290" distance of L0 L16
extrude "Extrude1''''" add sketch "Sketch1 (4)" against normal blind 2 separate body contours L0 L1 L3 L14 L21 L29 L31 | L1 L3 L14 L21 L30 L31 | L1 L2 L3 L21 L25 L30 L31 | A4 | A5 | A6 | A7 picked at (3.7724, -21.4514) picked at (-3.7724, 2.8486) picked at (-3.7724, 21.4514) picked at (12.7482, -17.3888) picked at (12.7355, 8.8345) picked at (-11.9518, -17.3888) picked at (-11.9645, 8.8345) makes body 4 in component "GM67"
extrude "Extrude2'''" add sketch "Sketch1 (4)" along normal blind 12 contours L0 L1 L3 L14 L15 L16 L17 L21 L29 L31 | L0 L1 L3 L14 L21 L29 L31 | A4 | A6 picked at (4.5833, -24.9167) picked at (3.7724, -21.4514) picked at (12.7482, -17.3888) picked at (-11.9518, -17.3888) bodies 4 in component "GM67"
move_body "Move1" bodies 4 to x (1, 0, 0) y (0, -1, 0) z (0, 0, -1) at (0, 0, 7.5) in component "GM67"
sketch "Sketch1 (5)" plane through (0, 0, 0) normal (0, 1, 0) x (1, 0, 0) in component "Trial printer"
  line L0 (36.75, 36.75) -> (-36.75, 36.75)
  line L1 (-36.75, 36.75) -> (-36.75, -36.75)
  line L2 (-36.75, -36.75) -> (36.75, -36.75)
  line L3 (36.75, -36.75) -> (36.75, 36.75)
  line L4 (36.75, 36.75) -> (-36.75, -36.75) construction
  line L5 (-36.75, 36.75) -> (36.75, -36.75) construction
  line L6 (46.75, 46.75) -> (-46.75, 46.75)
  line L7 (-46.75, 46.75) -> (-46.75, -46.75)
  line L8 (-46.75, -46.75) -> (46.75, -46.75)
  line L9 (46.75, -46.75) -> (46.75, 46.75)
  line L10 (-46.75, -46.75) -> (-46.75, -50.75)
  line L11 (-46.75, -50.75) -> (46.75, -50.75)
  line L12 (46.75, -50.75) -> (46.75, -46.75)
  line L13 (-46.75, 46.75) -> (-46.75, 50.75)
  line L14 (-46.75, 50.75) -> (46.75, 50.75)
  line L15 (46.75, 50.75) -> (46.75, 46.75)
  dimension "d357" = 73.5
  dimension "d358" = 73.5
  dimension "d359" = 10
  dimension "d360" = 10
  dimension "d361" = 10
  dimension "d362" = 10
  dimension "d363" = 4
  dimension "d364" = 4
  dimension "d390" = 101.5
  dimension "d391" = 93.5
  constraint horizontal L0
  constraint perpendicular L0 L1
  constraint parallel L0 L2
  constraint parallel L1 L3
  constraint coincident L4 origin
  constraint coincident L5 origin
  constraint horizontal L6
  constraint perpendicular L6 L7
  constraint parallel L6 L8
  constraint parallel L7 L9
  constraint perpendicular L8 L10
  constraint perpendicular L9 L11
  constraint perpendicular L8 L12
  constraint perpendicular L6 L13
  constraint perpendicular L9 L14
  constraint perpendicular L6 L15
  measures "d357" distance of L1.end L2.end
  measures "d358" distance of L0.end L1.end
  measures "d359" distance of L2 L8
  measures "d360" distance of L0 L6
  measures "d361" distance of L3 L9
  measures "d362" distance of L1 L7
  measures "d363" distance of L8 L11
  measures "d364" distance of L6 L14
  measures "d390" distance of L11 L14
  measures "d391" distance of L7 L9